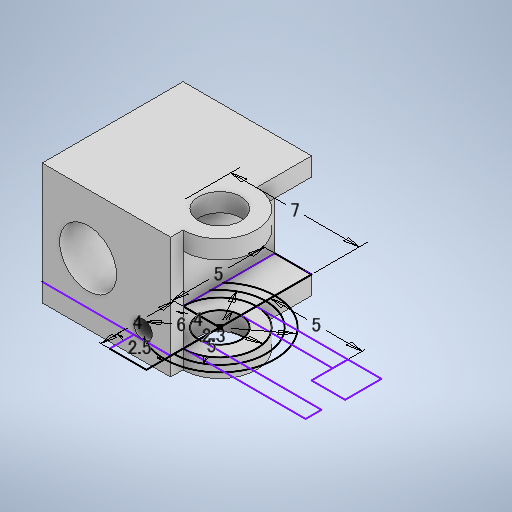
# Autodesk Inventor part: rod5.0
Saved by Autodesk Inventor 2025 (Build 290162000, 162)
## iProperties
Created: 2024-07-15
Part Number: rod5.0
Material: 一般
Document SubType Name: Modeling
Designer: Saigusa
Density: 1 g/cm^3
Appearance: 既定
Author: Saigusa
Autodesk Inventor part; units mm, degrees
ref_plane "YZ Plane" through (0, 0, 0) normal (1, 0, 0) x (0, 1, 0)
ref_plane "XZ Plane" through (0, 0, 0) normal (0, 1, 0) x (-1, 0, 0)
ref_plane "XY Plane" through (0, 0, 0) normal (0, 0, 1) x (1, 0, 0)
sketch "スケッチ1" plane through (0, 0, 0) normal (0, 1, 0) x (-1, 0, 0)
  circle A0 centre (0, 0) radius 2
  circle A1 centre (0, 0) radius 1.15
  line L0 (0, 0) -> (2, 0)
  line L1 (2, 0) -> (2, -5)
  line L2 (2, -5) -> (0, -5)
  line L3 (0, -5) -> (0, 0)
  line L4 (0, 0) -> (2, 0)
  line L5 (2, 0) -> (2, 4)
  line L6 (2, 4) -> (0, 4)
  line L7 (0, 4) -> (0, 0)
  circle A2 centre (0, 0) radius 3
  circle A3 centre (0, 0) radius 2.5
  line L8 (0, 0) -> (2.5, 0)
  line L9 (2.5, 0) -> (2.5, 2.6782)
  line L10 (2.5, 2.6782) -> (0, 2.6782)
  line L11 (0, 2.6782) -> (0, 0)
  line L12 (0, 2.6782) -> (7, 2.6782)
  line L13 (7, 2.6782) -> (7, -5)
  line L14 (7, -5) -> (0, -5)
  line L15 (0, -5) -> (0, 2.6782)
  point P0 (0, 2)
  point P1 (0, -2)
  dimension "d0" = 4
  dimension "d1" = 2.3
  dimension "d2" = 5
  dimension "d3" = 4
  dimension "d4" = 6
  dimension "d6" = 5
  dimension "d7" = 2.5
  dimension "d8" = 7
  constraints: 32 end point, 8 parallel, 4 centre point, 4 coincident, 4 horizontal, 4 perpendicular, 1 point on line
  measures "d0" diameter of A0
  measures "d1" diameter of A1
  measures "d2" distance of L0.end L1.end
  measures "d3" distance of L5.end L4.end
  measures "d4" diameter of A2
  measures "d6" diameter of A3
  measures "d7" distance of L10.end L9.end
  measures "d8" distance of L13.end L14.end
sketch "スケッチ2" plane through (0, 0, 0) normal (0, 1, 0) x (-1, 0, 0)
  line L0 (0, -1.1495) -> (-5, -1.1495)
  line L1 (-5, -1.1495) -> (-5, -1.9793)
  line L2 (-5, -1.9793) -> (0, -1.9793)
  line L3 (0, -1.9793) -> (0, -1.1495)
  line L4 (-5, -1.9793) -> (-6.828, -1.9793)
  line L5 (-6.828, -1.9793) -> (-6.828, 0)
  line L6 (-6.828, 0) -> (-5, 0)
  line L7 (-5, 0) -> (-5, -1.9793)
  line L8 (0, 1.115) -> (-6.6551, 1.115)
  line L9 (-6.6551, 1.115) -> (-6.6551, 1.9793)
  line L10 (-6.6551, 1.9793) -> (0, 1.9793)
  line L11 (0, 1.9793) -> (0, 1.115)
  point P0 (0, 0)
  dimension "d5" = 5
  constraints: 24 end point, 6 parallel, 3 horizontal, 3 perpendicular
  measures "d5" distance of L2.end L1.end
extrude "押し出し1" add sketch "スケッチ1" along normal blind 4.6 contours L8 A3 L1 | A0 L7 A3 L5 | L5 A3 L8 | A3 L9 A2 L1 | A3 L7 L10 A2 L5 | L5 A2 L9 A3 | A2 L9 L12 L13 L14 L1 | A2 L10 L5 | L5 L10 L9 A2
extrude "押し出し2" add sketch "スケッチ1" against normal blind 1 contours L0 A1 L7 A0 | L1 A3 L3 A0 | A0 L3 A1 L0 | L8 A3 L1 | A0 L7 A3 L5 | L5 A3 L8 | L7 A1 L3 A0 | A3 L9 A2 L1 | L1 A2 L3 A3 | A3 L7 L10 A2 L5 | L5 A2 L9 A3 | A2 L9 L12 L13 L14 L1 | L1 L2 L3 A2 | A2 L10 L5 | L5 L10 L9 A2
sketch "スケッチ3" plane through (0, 4.6, 0) normal (0, 1, 0) x (1, 0, 0)
  circle A0 centre (0, 0) radius 1.15
  line L0 (-2, 0) -> (-2, 5) projected
  circle A1 centre (0, 0) radius 2
  line L1 (0, -2) -> (0, -2.6782) projected
  line L2 (-7, 5) -> (0, 5) projected
  line L3 (0, -2.6782) -> (-7, -2.6782)
  line L4 (-7, -2.6782) -> (-7, 5)
  line L5 (-7, 5) -> (0, 5)
  line L6 (0, 5) -> (0, -2.6782)
  point P0 (0, 2)
  constraints: 8 end point, 2 centre point, 2 coincident, 2 parallel, 1 horizontal, 1 perpendicular, 1 point on circle
extrude "押し出し3" add sketch "スケッチ3" along normal blind 1 contours A0 L6 A1 | A0 L6 A1 | A1 L0 L2 L6 | L1 L3 L4 L2 L0 A1
sketch "スケッチ4" plane through (-7, -1, 2.6782) normal (0, 0, 1) x (1, 0, 0)
  line L0 (7, 6.6) -> (0, 6.6) projected
  line L1 (0, 6.6) -> (2.5, 6.6)
  line L2 (2.5, 6.6) -> (2.5, 3.35)
  line L3 (2.5, 3.35) -> (0, 3.35)
  line L4 (0, 3.35) -> (0, 6.6)
  circle A0 centre (2.5, 3.35) radius 1.55
  line L5 (5, 1) -> (7, 1) projected
  line L6 (7, 1) -> (5.5, 1)
  line L7 (5.5, 1) -> (5.5, 1.5)
  line L8 (5.5, 1.5) -> (7, 1.5)
  line L9 (7, 1.5) -> (7, 1)
  circle A1 centre (5.5, 1.5) radius 0.5
  dimension "d15" = 2.5
  dimension "d16" = 3.25
  dimension "d17" = 3.1
  dimension "d18" = 1.5
  dimension "d19" = 0.5
  constraints: 16 end point, 4 parallel, 2 centre point, 2 coincident, 2 horizontal, 2 perpendicular
  measures "d15" distance of L2.end L3.end
  measures "d16" distance of L1.end L2.end
  measures "d17" diameter of A0
  measures "d18" distance of L7.end L8.end
  measures "d19" distance of L6.end L7.end
extrude "押し出し4" cut sketch "スケッチ4" against normal blind 6 contours A0 L3 L2 | L2 L3 A0 | A1 L8 L7 | L7 L8 A1
